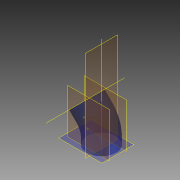
# Autodesk Inventor part: Ball Path
Saved by Autodesk Inventor 2014 SP1 (Build 180222100, 222)
## iProperties
Created: 2012-01-27
Part Number: Ball Path
Material: Generic
Document SubType Name: Modeling
Designer: Moses
Density: 1 g/cm^3
Mass: 204.895 g
Surface Area: 3242.8 cm^2
Volume: 204.895 cm^3
Appearance: Clear - Green 1
d14: 0.727 in
d15: 0.727 in
d17: 3.000 in
d18: 3.727 in
d19: 2.757 in
d20: 1.757 in
d21: 135.00 deg
d16: 0.727 in
Author: Moses
Autodesk Inventor part; units mm, degrees
ref_plane "XZ Plane" through (0, 0, 0) normal (0, 1, 0) x (-1, 0, 0)
sketch "Sketch1" plane through (0, 0, 0) normal (0, 0, 1) x (1, 0, 0)
  line L0 (0, 0) -> (0, 44.6369)
  line L1 (-22.3185, 98.5185) -> (-71.842, 148.042)
  arc A0 (0, 44.6369) -> (-22.3185, 98.5185) centre (-76.2, 44.6369) ccw
  point P0 (0, 76.2)
  dimension "d0" = 135
  dimension "d1" = 76.2
  dimension "d2" = 101.6
  dimension "d3" = 76.2
  constraints: 4 end point, 2 point on circle, 2 point on line, 2 tangent, 1 centre point, 1 vertical
  measures "d0" angle of L0 L1
  measures "d1" distance of L0.start point (0, 76.2)
  measures "d2" distance of point (0, 76.2) L1.end
  measures "d3" radius of A0
sketch "Sketch2" plane through (0, 0, 0) normal (0, 1, 0) x (-1, 0, 0)
  circle A0 centre (-101.6, 0) radius 101.6
  line L0 (0, 0) -> (-124.0253, 0) construction
  circle A1 centre (-101.6, 0) radius 100.33
  dimension "d4" = 203.2
  dimension "d6" = 1.27
  constraints: 2 end point, 1 centre point, 1 coincident, 1 horizontal, 1 horizontal alignment, 1 point on line, 2 other
sweep "Sweep1" add profiles "Sketch2" path "Sketch1"
ref_plane "Work Plane1" through (101.6, 0, 0) normal (1, 0, 0) x (0, 1, 0)
ref_plane "Work Plane4" through (101.6, 0, 0) normal (0, -1, 0) x (1, 0, 0)
ref_plane "Work Plane6" through (-71.842, 148.042, 0) normal (-0.7071, 0.7071, 0) x (-0.7071, -0.7071, 0)
ref_plane "Work Plane7" through (0, 0, 58.42) normal (0, 0, 1) x (1, 0, 0)
ref_plane "Work Plane8" through (0, 0, -58.42) normal (0, 0, 1) x (1, 0, 0)
sketch "Sketch4" plane through (0, 0, 58.42) normal (0, 0, 1) x (1, 0, 0)
  line L0 (58.7778, 278.6619) -> (108.3014, 229.1383) projected
  arc A0 (184.7244, 44.6369) -> (108.3014, 229.1383) centre (-76.2, 44.6369) ccw projected
  line L1 (184.7244, 44.6369) -> (184.7244, 0) projected
  line L2 (184.7244, 0) -> (183.1672, 0) projected
  line L3 (183.1672, 0) -> (183.1672, 44.6369) projected
  arc A1 (183.1672, 44.6369) -> (107.2003, 228.0373) centre (-76.2, 44.6369) ccw projected
  line L4 (107.2003, 228.0373) -> (57.6767, 277.5608) projected
  line L5 (57.6767, 277.5608) -> (58.7778, 278.6619) projected
  line L6 (-9.2542, 111.5827) -> (-58.7778, 161.1063) projected
  line L7 (-58.7778, 161.1063) -> (-57.6767, 162.2074) projected
  line L8 (-57.6767, 162.2074) -> (-8.1532, 112.6838) projected
  arc A2 (20.0328, 44.6369) -> (-8.1532, 112.6838) centre (-76.2, 44.6369) ccw projected
  line L9 (20.0328, 44.6369) -> (20.0328, 0) projected
  line L10 (20.0328, 0) -> (18.4756, 0) projected
  line L11 (18.4756, 0) -> (18.4756, 44.6369) projected
  arc A3 (18.4756, 44.6369) -> (-9.2542, 111.5827) centre (-76.2, 44.6369) ccw projected
  line L12 (-22.3185, 98.5185) -> (-71.842, 148.042) projected
  arc A4 (0, 44.6369) -> (-22.3185, 98.5185) centre (-76.2, 44.6369) ccw projected
  line L13 (0, 0) -> (0, 44.6369) projected
  line L14 (203.2, 0) -> (203.2, 44.6369) projected
  arc A5 (203.2, 44.6369) -> (121.3656, 242.2026) centre (-76.2, 44.6369) ccw projected
  line L15 (121.3656, 242.2026) -> (71.842, 291.7261) projected
  dimension "d14" = 18.4756
  dimension "d15" = 18.4756
  dimension "d16" = 18.4756
  dimension "d17" = 76.2
  dimension "d18" = 94.6756
  dimension "d19" = 70.0369
  dimension "d20" = 44.6369
  dimension "d21" = 135
  measures "d14" radial gap between concentric circles of A4 A3
  measures "d15" distance between parallel lines of L6 L12
  measures "d16" distance between parallel lines of L11 L13
  measures "d17" radius of A4
  measures "d18" radius of A3
  measures "d19" distance of L12.start L12.end
  measures "d20" distance of L13.start L13.end
  measures "d21" angle of L13 L12
equation "\"angle\" = 45deg"
equation "\"d8\" = -d7"
equation "\"d7\" = 58.42"
body "Solid1"
